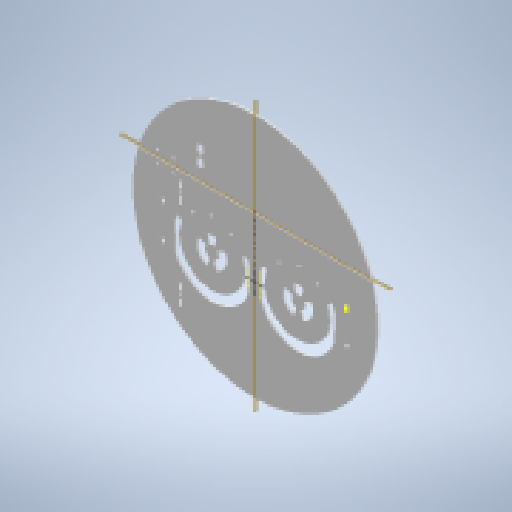
# Autodesk Inventor part: Деталь1
Saved by Autodesk Inventor 2023.2 (Build 272271030, 271C)
## iProperties
Created: 2024-01-26
Part Number: Деталь1
Material: Типовые
Document SubType Name: Modeling
Designer: I9232
Density: 1 g/cm^3
Appearance: По умолчанию
Author: I9232
Autodesk Inventor part; units mm, degrees
ref_plane "YZ Plane" through (0, 0, 0) normal (1, 0, 0) x (0, 1, 0)
ref_plane "XY Plane" through (0, 0, 0) normal (0, 0, 1) x (1, 0, 0)
sketch "Эскиз1" plane through (0, 0, 0) normal (0, 0, 1) x (1, 0, 0)
  circle A0 centre (-95.6307, 0) radius 127.844
  point P0 (0, 0)
  constraints: 1 centre point
extrude "Выдавливание1" add sketch "Эскиз1" along normal blind 2
sketch "Эскиз5" plane through (0, 0, 2) normal (0, 0, 1) x (1, 0, 0)
  circle A0 centre (-191.4705, -32.9366) radius 2 projected
  circle A1 centre (-191.4705, 2.9366) radius 2 projected
  circle A2 centre (0, 2.9366) radius 2 projected
  circle A3 centre (0, -32.9366) radius 2 projected
  circle A4 centre (-30.8327, 7.6483) radius 1.5 projected
  circle A5 centre (-50.2499, 14.2698) radius 1.5 projected
  circle A6 centre (-70.9883, 7.2463) radius 1.5 projected
  circle A7 centre (-120.4823, 7.2463) radius 1.5 projected
  circle A8 centre (-141.2206, 14.2698) radius 1.5 projected
  circle A9 centre (-160.6378, 7.6483) radius 1.5 projected
  arc A10 (-12.7161, -9.3219) -> (-16.1637, -1.7649) centre (-51.5496, -22.4733) ccw projected
  line L0 (-16.1637, -1.7649) -> (-20.1637, -6.3085) projected
  arc A11 (-82.9355, -5.4758) -> (-20.1637, -6.3085) centre (-51.725, -19.1185) ccw projected
  line L1 (-82.9355, -5.4758) -> (-88.8603, -5.4758) projected
  arc A12 (-88.8603, -5.4758) -> (-90.3831, -9.3219) centre (-51.5496, -22.4733) ccw projected
  line L2 (-90.3831, -9.3219) -> (-89.9328, -36.8861) projected
  arc A13 (-89.9328, -36.8861) -> (-13.1664, -36.8861) centre (-51.5496, -22.4733) ccw projected
  line L3 (-13.1664, -36.8861) -> (-12.7161, -9.3219) projected
  line L4 (-179.4162, -9.3219) -> (-178.9659, -36.8861) projected
  arc A14 (-178.9659, -36.8861) -> (-102.1995, -36.8861) centre (-140.5827, -22.4733) ccw projected
  line L5 (-102.1995, -36.8861) -> (-101.7492, -9.3219) projected
  arc A15 (-101.7492, -9.3219) -> (-103.2721, -5.4758) centre (-140.5827, -22.4733) ccw projected
  line L6 (-103.2721, -5.4758) -> (-109.1968, -6.3085) projected
  arc A16 (-171.9686, -6.3085) -> (-109.1968, -6.3085) centre (-140.5827, -19.1724) ccw projected
  line L7 (-171.9686, -6.3085) -> (-175.9686, -1.7649) projected
  arc A17 (-175.9686, -1.7649) -> (-179.4162, -9.3219) centre (-140.5827, -22.4733) ccw projected
  arc A18 (-45.6461, -4.0105) -> (-55.6209, -4) centre (-50.6489, -18.6809) ccw projected
  line L8 (-55.6209, -4) -> (-53.8449, -12.3024) projected
  arc A19 (-47.4855, -12.1853) -> (-53.8449, -12.3024) centre (-50.5504, -18.4786) ccw projected
  line L9 (-47.4855, -12.1853) -> (-45.6461, -4.0105) projected
  line L10 (-137.6256, -12.3024) -> (-135.8496, -4) projected
  arc A20 (-135.8496, -4) -> (-145.8244, -4.0105) centre (-140.8216, -18.6809) ccw projected
  line L11 (-145.8244, -4.0105) -> (-143.985, -12.1853) projected
  arc A21 (-137.6256, -12.3024) -> (-143.985, -12.1853) centre (-140.9201, -18.4786) ccw projected
  arc A22 (-135.8665, -33.3675) -> (-126.822, -12.0281) centre (-140.8216, -18.6809) ccw projected
  line L12 (-126.822, -12.0281) -> (-135.0144, -14.7207) projected
  arc A23 (-138.9215, -25.1872) -> (-135.0144, -14.7207) centre (-140.9201, -18.4786) ccw projected
  line L13 (-138.9215, -25.1872) -> (-135.8665, -33.3675) projected
  arc A24 (-64.6485, -12.0281) -> (-55.604, -33.3675) centre (-50.6489, -18.6809) ccw projected
  line L14 (-55.604, -33.3675) -> (-52.549, -25.1872) projected
  arc A25 (-56.4561, -14.7207) -> (-52.549, -25.1872) centre (-50.5504, -18.4786) ccw projected
  line L15 (-56.4561, -14.7207) -> (-64.6485, -12.0281) projected
  arc A26 (-45.6939, -33.3676) -> (-36.6645, -11.9961) centre (-50.6489, -18.6809) ccw projected
  line L16 (-36.6645, -11.9961) -> (-44.6776, -14.6694) projected
  arc A27 (-48.7266, -25.2369) -> (-44.6776, -14.6694) centre (-50.5504, -18.4786) ccw projected
  line L17 (-48.7266, -25.2369) -> (-45.6939, -33.3676) projected
  arc A28 (-146.793, -14.6694) -> (-142.7439, -25.2369) centre (-140.9201, -18.4786) ccw projected
  line L18 (-146.793, -14.6694) -> (-154.806, -11.9961) projected
  arc A29 (-154.806, -11.9961) -> (-145.7766, -33.3676) centre (-140.8216, -18.6809) ccw projected
  line L19 (-145.7766, -33.3676) -> (-142.7439, -25.2369) projected
  point P0 (0, 0)
extrude "Выдавливание5" cut sketch "Эскиз5" against normal blind 2
sketch "Эскиз11" plane through (-95.6307, 0, 2) normal (0, 0, 1) x (1, 0, 0)
  line L0 (-6.5688, -36.8861) -> (-6.1185, -9.3219) construction
  line L1 (-6.3437, -23.104) -> (5.4727, -23.104) construction
  line L2 (5.6979, -36.8861) -> (5.2476, -9.3219) construction
  line L3 (-0.4355, 43.8357) -> (-0.4355, -36.6138) construction
  point P0 (95.6307, 0)
  point P1 (-0.4355, -23.104)
  constraints: 4 end point, 3 midpoint, 1 point on line, 1 vertical
ref_plane "Плоскость центральной симметрии" through (-96.0662, 43.8357, 2) normal (-1, 0, 0) x (0, -1, 0)
sketch "Эскиз8" plane through (0, 0, 2) normal (0, 0, 1) x (1, 0, 0)
  circle A0 centre (-197.0662, 33) radius 1.25
  circle A1 centre (-181.0662, 33) radius 1.25
  line L0 (-96.0662, -178.9816) -> (-96.0662, 178.9816) projected
  line L1 (-181.0662, 33) -> (-197.0662, 33) construction
  circle A2 centre (-181.0662, 46.028) radius 1.25
  circle A3 centre (-197.0662, 46.028) radius 1.25
  point P0 (0, 0)
  dimension "d23" = 85
  dimension "d24" = 16
  dimension "d25" = 33
  dimension "d26" = 2.5
  dimension "d29" = 13.028
  constraints: 4 centre point, 2 end point, 1 equal radius, 1 horizontal, 1 vertical, 4 other
  measures "d23" distance from line of L1.start L0
  measures "d24" distance of L1.end L1.start
  measures "d25" vertical distance of L1.start point (0, 0)
  measures "d26" diameter of A1
  measures "d29" distance of L1.start A2.centre
extrude "Выдавливание8" cut sketch "Эскиз8" against normal blind 2
sketch "Эскиз9" plane through (0, 0, 2) normal (0, 0, 1) x (1, 0, 0)
  point P0 (0, 0)
ref_plane "РабПлоскость2" through (0, 40, 0) normal (0, 1, 0) x (-1, 0, 0)
split body "Разделение2" result two bodies by plane through (0, 40, 0) normal (0, 1, 0) first body at (-44.6289, 46.6318, 0.5)
sketch "Эскиз3" plane through (-95.6307, 0, 2) normal (0, 0, 1) x (1, 0, 0)
  circle A0 centre (0, 0) radius 127.844 projected
  line L0 (121.9057, 38.5109) -> (-121.9057, 38.5109)
  line L1 (121.35, 40.2278) -> (-121.35, 40.2278)
  arc A1 (-121.35, 40.2278) -> (-121.9057, 38.5109) centre (0, 0) ccw
  arc A2 (121.9057, 38.5109) -> (121.35, 40.2278) centre (0, 0) ccw
  point P0 (95.6307, 0)
  constraints: 8 point on circle, 4 end point, 2 centre point, 1 concentric, 1 horizontal, 1 parallel
extrude "Выдавливание3" cut sketch "Эскиз3" against normal blind 2 contours L0 A0 L1 bodies 2 3
sketch "Эскиз12" plane through (0, 0, 2) normal (0, 0, 1) x (1, 0, 0)
  line L0 (-171.3841, -62.723) -> (-174.3841, -62.723) projected
  line L1 (-174.3841, -62.723) -> (-174.3841, -69.723) projected
  line L2 (-174.3841, -69.723) -> (-171.3841, -69.723) projected
  line L3 (-171.3841, -69.723) -> (-171.3841, -62.723) projected
  line L4 (-171.3841, -76.723) -> (-174.3841, -76.723) projected
  line L5 (-174.3841, -76.723) -> (-174.3841, -83.723) projected
  line L6 (-174.3841, -83.723) -> (-171.3841, -83.723) projected
  line L7 (-171.3841, -83.723) -> (-171.3841, -76.723) projected
  line L8 (-171.3841, 15.777) -> (-174.3841, 15.777) projected
  line L9 (-174.3841, 15.777) -> (-174.3841, 8.777) projected
  line L10 (-174.3841, 8.777) -> (-171.3841, 8.777) projected
  line L11 (-171.3841, 8.777) -> (-171.3841, 15.777) projected
  line L12 (-171.3841, 29.777) -> (-174.3841, 29.777) projected
  line L13 (-174.3841, 29.777) -> (-174.3841, 22.777) projected
  line L14 (-174.3841, 22.777) -> (-171.3841, 22.777) projected
  line L15 (-171.3841, 22.777) -> (-171.3841, 29.777) projected
  line L16 (-172.8841, -69.723) -> (-172.8841, -76.723) construction
  line L17 (-172.8841, 22.777) -> (-172.8841, 15.777) construction
  circle A0 centre (-172.8841, -73.223) radius 1.25
  circle A1 centre (-172.8841, 19.277) radius 1.25
  point P0 (0, 0)
  constraints: 6 midpoint, 4 end point, 2 centre point, 1 equal radius
extrude "Выдавливание10" cut sketch "Эскиз12" against normal through all bodies 3
sketch "Эскиз13" plane through (0, 0, 0) normal (0, 0, -1) x (-1, 0, 0)
  line L0 (170.9974, 65.7571) -> (164.9974, 65.7571) construction
  line L1 (164.9974, 65.7571) -> (164.9974, 85.7571) construction
  line L2 (164.9974, 85.7571) -> (170.9974, 85.7571) construction
  line L3 (170.9974, 85.7571) -> (170.9974, 65.7571) construction
  line L4 (170.9974, 65.7571) -> (164.9974, 65.7571)
  line L5 (164.9974, 65.7571) -> (164.9974, 72.7571)
  line L6 (164.9974, 72.7571) -> (170.9974, 72.7571)
  line L7 (170.9974, 72.7571) -> (170.9974, 65.7571)
  line L8 (170.9974, 75.7571) -> (164.9974, 75.7571) construction
  line L9 (170.9974, 85.7571) -> (164.9974, 85.7571) construction
  line L10 (170.9974, 85.7571) -> (164.9974, 85.7571)
  line L11 (164.9974, 85.7571) -> (164.9974, 78.7571)
  line L12 (164.9974, 78.7571) -> (170.9974, 78.7571)
  line L13 (170.9974, 78.7571) -> (170.9974, 85.7571)
  point P0 (0, 0)
  dimension "d37" = 6
  dimension "d38" = 20
  dimension "d39" = 7
  constraints: 28 end point, 4 parallel, 4 symmetric about line, 2 horizontal, 2 midpoint, 2 perpendicular, 1 point on line
  measures "d37" distance of L8.start L8.end
  measures "d38" distance of L2.end L0.start
  measures "d39" distance between parallel lines of L0 L6
extrude "Выдавливание11" cut sketch "Эскиз13" against normal through all bodies 2
